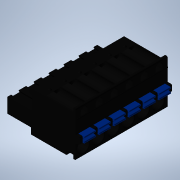
# Autodesk Inventor part: 8079509 6GD-1RR5,08-CLP-CBL
Saved by Autodesk Inventor 2021 (Build 250183000, 183)
## iProperties
Created: 2026-04-23
Part Number: 8079509 6GD-1RR5,08-CLP-CBL
Material: Generic
Catalog Web Link: www.3dfindit.com
Description: NEKM-C6 (p)-terminal strip
Vendor: FESTO
Document SubType Name: Modeling
Designer: psAdmin
Manufacturer: FESTO
Mass: 7.38948 g
Surface Area: 41.4115 cm^2
Volume: 7.38948 cm^3
Density: 1 g/cm^3
Appearance: PSOLRGB-80-80-80
Category: PARTsolutions
Company: FESTO
Title: 8079509 6GD-1RR5,08-CLP-CBL
Author: Cadenas PARTsolutions
Comments: terminal strip
PSOL_IDENT_0: {$CADENAS_DATA/23d-libs/festo/parts/n/nekm/parts/nekm_c6_parts.prj},200 {VTYP=3D},{NB=8079509 6GD-1R
PSOL_IDENT_1: R5,08-CLP-CBL},{LINA=8079509 6GD-1RR5,08-CLP-CBL},{NN=NEKM-C6 (p)},{DATE=26.08.2025 07:05:50},{GEOMD
PSOL_IDENT_2: ATE=26.08.2025 07:05:00},{VERSION=},{LINEID=170},{WBVAR=},{WBNUMERIC=}  {NB=8079509 6GD-1RR5,08-CLP-
PSOL_IDENT_3: CBL},{LINA=8079509 6GD-1RR5,08-CLP-CBL},{KT=DUMMY},{TNR=8079509},{TYP=6GD-1RR5,08-CLP-CBL},{VERS=2},
PSOL_IDENT_4: {N=6},{L=31.100},{L1=3.790}
NB: 8079509 6GD-1RR5,08-CLP-CBL
NN: NEKM-C6 (p)
NT: terminal strip
NBSYN: $TNR. $TYP.
LINA: 8079509 6GD-1RR5,08-CLP-CBL
CATALOG: Festo
TNR: 8079509
TYP: 6GD-1RR5,08-CLP-CBL
VERS: 2
N: 6
L: 31.1
L1: 3.79
SUPPLIER: FESTO
ARTICLENO: 8079509 6GD-1RR5,08-CLP-CBL
BOMINFO: 8079509 6GD-1RR5,08-CLP-CBL
CREATOR: CADENAS GmbH
Autodesk Inventor part; units mm, degrees
sketch "Sketch_1" plane through (0, 0, 0) normal (0, 0, 1) x (1, 0, 0)
  line L0 (0, 6) -> (0, -7.5)
  line L1 (0, -7.5) -> (14.43, -7.5)
  arc A0 (14.43, -7.5) -> (14.73, -7.2) centre (14.43, -7.2) ccw
  line L2 (14.73, -7.2) -> (14.73, 4.1)
  arc A1 (14.73, 4.1) -> (14.73, 4.5) centre (14.73, 4.3) ccw
  line L3 (14.73, 4.5) -> (14.73, 7.2)
  arc A2 (14.73, 7.2) -> (14.43, 7.5) centre (14.43, 7.2) ccw
  line L4 (14.43, 7.5) -> (13.93, 7.5)
  line L5 (13.93, 7.5) -> (13.93, 6)
  line L6 (13.93, 6) -> (0, 6)
  constraints: 14 end point, 6 point on circle, 3 centre point
extrude "Extrusion1" add sketch "Sketch_1" along normal mid plane 31.1
sketch "Sketch_2" plane through (0, 0, 15.55) normal (0, 0, 1) x (1, 0, 0)
  line L0 (14.73, 0.2) -> (14.73, -2.856)
  arc A0 (14.9274, -2.5741) -> (14.73, -2.856) centre (15.03, -2.856) ccw
  line L1 (14.9274, -2.5741) -> (16.0326, -2.1718)
  arc A1 (16.0326, -2.1718) -> (16.23, -1.8899) centre (15.93, -1.8899) ccw
  line L2 (16.23, -1.8899) -> (16.23, -0.3)
  arc A2 (16.23, -0.3) -> (15.93, 0) centre (15.93, -0.3) ccw
  line L3 (15.93, 0) -> (14.93, 0)
  arc A3 (14.73, 0.2) -> (14.93, 0) centre (14.93, 0.2) ccw
  constraints: 8 end point, 8 point on circle, 4 centre point
extrude "Extrusion2" add sketch "Sketch_2" against normal blind 0.8
pattern_linear "Rectangular Pattern1" count 2 spacing 30.3 along (0, 0, -1) of "Extrusion2"
sketch "Sketch_4" plane through (0, 0, 10.65) normal (0, 0, 1) x (1, 0, 0)
  line L0 (14.73, 0.2) -> (14.73, -2.756)
  arc A0 (14.9274, -2.4741) -> (14.73, -2.756) centre (15.03, -2.756) ccw
  line L1 (14.9274, -2.4741) -> (16.0326, -2.0718)
  arc A1 (16.0326, -2.0718) -> (16.23, -1.7899) centre (15.93, -1.7899) ccw
  line L2 (16.23, -1.7899) -> (16.23, -0.3)
  arc A2 (16.23, -0.3) -> (15.93, 0) centre (15.93, -0.3) ccw
  line L3 (15.93, 0) -> (14.93, 0)
  arc A3 (14.73, 0.2) -> (14.93, 0) centre (14.93, 0.2) ccw
  constraints: 8 end point, 8 point on circle, 4 centre point
extrude "Extrusion3" add sketch "Sketch_4" against normal blind 0.98
pattern_linear "Rectangular Pattern2" count 5 spacing 5.08 along (0, 0, -1) of "Extrusion3"
sketch "Sketch_6" plane through (0, 0, 14.65) normal (0, 0, 1) x (1, 0, 0)
  line L0 (14.73, -2.075) -> (16.6, -2.075)
  arc A0 (16.6, -2.075) -> (16.8, -1.875) centre (16.6, -1.875) ccw
  line L1 (16.8, -1.875) -> (16.8, -1.7601)
  arc A1 (16.8, -1.7601) -> (16.6041, -1.516) centre (16.55, -1.7601) ccw
  line L2 (16.6041, -1.516) -> (15.9359, -1.3679)
  arc A2 (15.9359, -0.7821) -> (15.9359, -1.3679) centre (16.0008, -1.075) ccw
  line L3 (15.9359, -0.7821) -> (16.6041, -0.634)
  arc A3 (16.6041, -0.634) -> (16.8, -0.3899) centre (16.55, -0.3899) ccw
  line L4 (16.8, -0.3899) -> (16.8, -0.275)
  arc A4 (16.8, -0.275) -> (16.6, -0.075) centre (16.6, -0.275) ccw
  line L5 (16.6, -0.075) -> (14.73, -0.075)
  line L6 (14.73, -0.075) -> (14.73, -2.075)
  constraints: 14 end point, 10 point on circle, 5 centre point
extrude "Extrusion4" add sketch "Sketch_6" against normal blind 3.9
pattern_linear "Rectangular Pattern3" count 6 spacing 5.08 along (0, 0, -1) of "Extrusion4"
sketch "Sketch_8" plane through (0, -4.65, 0) normal (0, 1, 0) x (1, 0, 0)
  line L0 (14.73, -12.9) -> (11.73, -12.9)
  line L1 (11.73, -12.9) -> (11.73, -10.9)
  line L2 (11.73, -10.9) -> (14.53, -10.9)
  arc A0 (14.53, -10.9) -> (14.73, -10.7) centre (14.53, -10.7) ccw
  line L3 (14.73, -10.7) -> (14.73, -12.9)
  line L4 (14.73, -12.9) -> (11.73, -12.9)
  constraints: 10 end point, 2 point on circle, 1 centre point
revolve "Revolution1" cut sketch "Sketch_8" angle 360 about axis through (14.73, -4.65, 12.9) along (1, 0, 0)
pattern_linear "Rectangular Pattern4" count 6 spacing 5.08 along (0, 0, -1) of "Revolution1"
sketch "Sketch_10" plane through (13.93, 0, 0) normal (1, 0, 0) x (0, 0, -1)
  line L0 (-14.9913, 6) -> (-10.4087, 6)
  arc A0 (-10.4087, 6) -> (-14.9913, 6) centre (-12.7, 5) ccw
  constraints: 2 end point, 2 point on circle, 1 centre point
extrude "Extrusion5" add sketch "Sketch_10" against normal blind 9.7
pattern_linear "Rectangular Pattern5" count 6 spacing 5.08 along (0, 0, -1) of "Extrusion5"
sketch "Sketch_12" plane through (0, 0, 0) normal (0, 0, 1) x (1, 0, 0)
  line L0 (2, 7.5) -> (2, 6)
  line L1 (2, 6) -> (4.23, 6)
  line L2 (4.23, 6) -> (5.73, 7.5)
  line L3 (5.73, 7.5) -> (2, 7.5)
  constraints: 8 end point
extrude "Extrusion6" cut sketch "Sketch_12" along normal mid plane 31.1
sketch "Sketch_13" plane through (14.73, 0, 0) normal (1, 0, 0) x (0, 0, -1)
  line L0 (-13.875, 5.775) -> (-13.875, 4.6)
  line L1 (-13.875, 4.6) -> (-11.525, 4.6)
  line L2 (-11.525, 4.6) -> (-11.525, 5.775)
  arc A0 (-11.525, 5.775) -> (-13.875, 5.775) centre (-12.7, 5.775) ccw
  constraints: 6 end point, 2 point on circle, 1 centre point
extrude "Extrusion7" cut sketch "Sketch_13" against normal blind 9.325
pattern_linear "Rectangular Pattern6" count 6 spacing 5.08 along (0, 0, -1) of "Extrusion7"
sketch "Sketch_15" plane through (0, 7.5, 0) normal (0, 1, 0) x (1, 0, 0)
  arc A0 (5.405, -11.525) -> (5.405, -13.875) centre (5.405, -12.7) ccw
  line L0 (5.405, -13.875) -> (6.58, -13.875)
  line L1 (6.58, -13.875) -> (6.58, -11.525)
  line L2 (6.58, -11.525) -> (5.405, -11.525)
  constraints: 6 end point, 2 point on circle, 1 centre point
extrude "Extrusion8" cut sketch "Sketch_15" against normal blind 2.9
pattern_linear "Rectangular Pattern7" count 6 spacing 5.08 along (0, 0, -1) of "Extrusion8"
sketch "Sketch_17" plane through (3.13, 0, 0) normal (1, 0, 0) x (0, 0, -1)
  line L0 (-12.7, 6) -> (-12.7, 6.3)
  arc A0 (-12.25, 6) -> (-12.7, 6.3) centre (-12.7083, 5.8001) ccw
  line L1 (-12.25, 6) -> (-12.7, 6)
  line L2 (-12.7, 6) -> (-12.7, 6.3)
  constraints: 6 end point, 2 point on circle, 1 centre point
revolve "Revolution2" add sketch "Sketch_17" angle 360 about axis through (3.13, 6, 12.7) along (0, -1, 0)
pattern_linear "Rectangular Pattern8" count 6 spacing 5.08 along (0, 0, -1) of "Revolution2"
sketch "Sketch_25" plane through (0, 0, 0) normal (0, 0, 1) x (1, 0, 0)
  line L0 (-0.5, -0.795) -> (-0.5, -7.5)
  line L1 (-0.5, -7.5) -> (0, -7.5)
  line L2 (0, -7.5) -> (0, 0.071)
  line L3 (0, 0.071) -> (-0.5, -0.795)
  constraints: 8 end point
extrude "Extrusion9" add sketch "Sketch_25" along normal mid plane 31.1
sketch "Sketch_37" plane through (-0.5, 0, 0) normal (1, 0, 0) x (0, 0, -1)
  line L0 (-15.24, -5.71) -> (-14.8207, -5.71)
  arc A0 (-14.8207, -5.71) -> (-10.5793, -5.71) centre (-12.7, -3.71) ccw
  line L1 (-10.5793, -5.71) -> (-9.7407, -5.71)
  arc A1 (-9.7407, -5.71) -> (-5.4993, -5.71) centre (-7.62, -3.71) ccw
  line L2 (-5.4993, -5.71) -> (-4.6607, -5.71)
  arc A2 (-4.6607, -5.71) -> (-0.4193, -5.71) centre (-2.54, -3.71) ccw
  line L3 (-0.4193, -5.71) -> (0.4193, -5.71)
  arc A3 (0.4193, -5.71) -> (4.6607, -5.71) centre (2.54, -3.71) ccw
  line L4 (4.6607, -5.71) -> (5.4993, -5.71)
  arc A4 (5.4993, -5.71) -> (9.7407, -5.71) centre (7.62, -3.71) ccw
  line L5 (9.7407, -5.71) -> (10.5793, -5.71)
  arc A5 (10.5793, -5.71) -> (14.8207, -5.71) centre (12.7, -3.71) ccw
  line L6 (14.8207, -5.71) -> (15.24, -5.71)
  line L7 (15.24, -5.71) -> (15.24, -0.795)
  line L8 (15.24, -0.795) -> (13.957, -0.795)
  line L9 (13.957, -0.795) -> (14.3496, -1.475)
  line L10 (14.3496, -1.475) -> (11.0534, -1.475)
  line L11 (11.0534, -1.475) -> (11.446, -0.795)
  line L12 (11.446, -0.795) -> (8.877, -0.795)
  line L13 (8.877, -0.795) -> (9.2696, -1.475)
  line L14 (9.2696, -1.475) -> (5.9734, -1.475)
  line L15 (5.9734, -1.475) -> (6.366, -0.795)
  line L16 (6.366, -0.795) -> (3.797, -0.795)
  line L17 (3.797, -0.795) -> (4.1896, -1.475)
  line L18 (4.1896, -1.475) -> (0.8934, -1.475)
  line L19 (0.8934, -1.475) -> (1.286, -0.795)
  line L20 (1.286, -0.795) -> (-1.283, -0.795)
  line L21 (-1.283, -0.795) -> (-0.8904, -1.475)
  line L22 (-0.8904, -1.475) -> (-4.1866, -1.475)
  line L23 (-4.1866, -1.475) -> (-3.794, -0.795)
  line L24 (-3.794, -0.795) -> (-6.363, -0.795)
  line L25 (-6.363, -0.795) -> (-5.9704, -1.475)
  line L26 (-5.9704, -1.475) -> (-9.2666, -1.475)
  line L27 (-9.2666, -1.475) -> (-8.874, -0.795)
  line L28 (-8.874, -0.795) -> (-11.443, -0.795)
  line L29 (-11.443, -0.795) -> (-11.0504, -1.475)
  line L30 (-11.0504, -1.475) -> (-14.3466, -1.475)
  line L31 (-14.3466, -1.475) -> (-13.954, -0.795)
  line L32 (-13.954, -0.795) -> (-15.24, -0.795)
  line L33 (-15.24, -0.795) -> (-15.24, -5.71)
  constraints: 68 end point, 12 point on circle, 6 centre point
extrude "Extrusion10" add sketch "Sketch_37" against normal blind 8.3
sketch "Sketch13" plane through (-8.8, 0, 0) normal (-1, 0, 0) x (0, 0, 1)
  point P0 (12.7, -3.71)
hole "Hole1" at (-8.8, -3.71, 12.7) direction (1, 0, 0) diameter 1.4 depth 2 counterbore diameter 2.8 counterbore depth 1
pattern_linear "Rectangular Pattern9" count 6 spacing 5.08 along (0, 0, -1) of "Hole1"
sketch "Sketch_30" plane through (0, 0, 11.76) normal (0, 0, 1) x (1, 0, 0)
  arc A0 (-4.9014, 1.2616) -> (-4.86, 0.947) centre (-4.76, 1.1202) ccw
  line L0 (-4.86, 0.947) -> (-4.1642, 0.5453)
  arc A1 (-4.1642, 0.5453) -> (-3.8021, 0.5929) centre (-4.0142, 0.8051) ccw
  line L1 (-3.8021, 0.5929) -> (-3.53, 0.865)
  line L2 (-3.53, 0.865) -> (-0.3256, 1.0049)
  arc A2 (-0.3, 0.406) -> (-0.3256, 1.0049) centre (-0.3, 0.706) ccw
  arc A3 (-0.3, 0.406) -> (-0.5, 0.206) centre (-0.3, 0.206) ccw
  line L3 (-0.5, 0.206) -> (-0.5, -1)
  line L4 (-0.5, -1) -> (0.5, -1)
  line L5 (0.5, -1) -> (0.5, 3.3534)
  line L6 (0.5, 3.3534) -> (0, 3.3534)
  arc A4 (-0.2325, 3.0611) -> (0, 3.3534) centre (-0.3, 3.3534) ccw
  line L7 (-0.2325, 3.0611) -> (-3.7536, 2.2482)
  arc A5 (-3.7536, 2.2482) -> (-4.1152, 2.0478) centre (-3.5849, 1.5174) ccw
  line L8 (-4.1152, 2.0478) -> (-4.9014, 1.2616)
  constraints: 18 end point, 12 point on circle, 6 centre point
extrude "Extrusion11" add sketch "Sketch_30" against normal blind 1.6
sketch "Sketch_31" plane through (0, 0, -11.76) normal (0, 0, 1) x (1, 0, 0)
  arc A0 (-4.9014, 1.2616) -> (-4.86, 0.947) centre (-4.76, 1.1202) ccw
  line L0 (-4.86, 0.947) -> (-4.1642, 0.5453)
  arc A1 (-4.1642, 0.5453) -> (-3.8021, 0.5929) centre (-4.0142, 0.8051) ccw
  line L1 (-3.8021, 0.5929) -> (-3.53, 0.865)
  line L2 (-3.53, 0.865) -> (-0.3256, 1.0049)
  arc A2 (-0.3, 0.406) -> (-0.3256, 1.0049) centre (-0.3, 0.706) ccw
  arc A3 (-0.3, 0.406) -> (-0.5, 0.206) centre (-0.3, 0.206) ccw
  line L3 (-0.5, 0.206) -> (-0.5, -1)
  line L4 (-0.5, -1) -> (0.5, -1)
  line L5 (0.5, -1) -> (0.5, 3.3534)
  line L6 (0.5, 3.3534) -> (0, 3.3534)
  arc A4 (-0.2325, 3.0611) -> (0, 3.3534) centre (-0.3, 3.3534) ccw
  line L7 (-0.2325, 3.0611) -> (-3.7536, 2.2482)
  arc A5 (-3.7536, 2.2482) -> (-4.1152, 2.0478) centre (-3.5849, 1.5174) ccw
  line L8 (-4.1152, 2.0478) -> (-4.9014, 1.2616)
  constraints: 18 end point, 12 point on circle, 6 centre point
extrude "Extrusion12" add sketch "Sketch_31" along normal blind 1.6
sketch "Sketch_39" plane through (11.58, 0, 0) normal (1, 0, 0) x (0, 0, -1)
  line L0 (-15.55, -8.25) -> (15.55, -8.25)
  line L1 (15.55, -8.25) -> (15.55, -6.25)
  line L2 (15.55, -6.25) -> (14.8585, -6.25)
  arc A0 (10.1415, -6.25) -> (14.8585, -6.25) centre (12.5, -4.65) ccw
  line L3 (10.1415, -6.25) -> (9.7785, -6.25)
  arc A1 (5.0615, -6.25) -> (9.7785, -6.25) centre (7.42, -4.65) ccw
  line L4 (5.0615, -6.25) -> (4.6985, -6.25)
  arc A2 (-0.0185, -6.25) -> (4.6985, -6.25) centre (2.34, -4.65) ccw
  line L5 (-0.0185, -6.25) -> (-0.3815, -6.25)
  arc A3 (-5.0985, -6.25) -> (-0.3815, -6.25) centre (-2.74, -4.65) ccw
  line L6 (-5.0985, -6.25) -> (-5.4615, -6.25)
  arc A4 (-10.1785, -6.25) -> (-5.4615, -6.25) centre (-7.82, -4.65) ccw
  line L7 (-10.1785, -6.25) -> (-10.5415, -6.25)
  arc A5 (-15.2585, -6.25) -> (-10.5415, -6.25) centre (-12.9, -4.65) ccw
  line L8 (-15.2585, -6.25) -> (-15.55, -6.25)
  line L9 (-15.55, -6.25) -> (-15.55, -8.25)
  constraints: 20 end point, 12 point on circle, 6 centre point
extrude "Extrusion13" cut sketch "Sketch_39" along normal blind 2.35
ref_plane "ANBAU_XY" through (0, 0, 0) normal (0, 1, 0) x (1, 0, 0)
ref_plane "ANBAU_YZ" through (0, 0, 0) normal (1, 0, 0) x (0, 0, -1)
ref_plane "ANBAU_ZX" through (0, 0, 0) normal (0, 0, -1) x (0, 1, 0)
ref_plane "CP1_XY" through (-0.5, -3.71, 0) normal (1, 0, 0) x (0, 0, -1)
ref_plane "CP1_YZ" through (-0.5, -3.71, 0) normal (0, 0, -1) x (0, 1, 0)
ref_plane "CP1_ZX" through (-0.5, -3.71, 0) normal (0, 1, 0) x (1, 0, 0)
ref_plane "ECP_1_XY" through (2.73, -4.65, 12.9) normal (1, 0, 0) x (0, 0, -1)
ref_plane "ECP_1_YZ" through (2.73, -4.65, 12.9) normal (0, 0, -1) x (0, 1, 0)
ref_plane "ECP_1_ZX" through (2.73, -4.65, 12.9) normal (0, 1, 0) x (1, 0, 0)
ref_plane "ECP_2_XY" through (2.73, -4.65, 7.82) normal (1, 0, 0) x (0, 0, -1)
ref_plane "ECP_2_YZ" through (2.73, -4.65, 7.82) normal (0, 0, -1) x (0, 1, 0)
ref_plane "ECP_2_ZX" through (2.73, -4.65, 7.82) normal (0, 1, 0) x (1, 0, 0)
ref_plane "ECP_3_XY" through (2.73, -4.65, 2.74) normal (1, 0, 0) x (0, 0, -1)
ref_plane "ECP_3_YZ" through (2.73, -4.65, 2.74) normal (0, 0, -1) x (0, 1, 0)
ref_plane "ECP_3_ZX" through (2.73, -4.65, 2.74) normal (0, 1, 0) x (1, 0, 0)
ref_plane "ECP_4_XY" through (2.73, -4.65, -2.34) normal (1, 0, 0) x (0, 0, -1)
ref_plane "ECP_4_YZ" through (2.73, -4.65, -2.34) normal (0, 0, -1) x (0, 1, 0)
ref_plane "ECP_4_ZX" through (2.73, -4.65, -2.34) normal (0, 1, 0) x (1, 0, 0)
ref_plane "ECP_5_XY" through (2.73, -4.65, -7.42) normal (1, 0, 0) x (0, 0, -1)
ref_plane "ECP_5_YZ" through (2.73, -4.65, -7.42) normal (0, 0, -1) x (0, 1, 0)
ref_plane "ECP_5_ZX" through (2.73, -4.65, -7.42) normal (0, 1, 0) x (1, 0, 0)
ref_plane "ECP_6_XY" through (2.73, -4.65, -12.5) normal (1, 0, 0) x (0, 0, -1)
ref_plane "ECP_6_YZ" through (2.73, -4.65, -12.5) normal (0, 0, -1) x (0, 1, 0)
ref_plane "ECP_6_ZX" through (2.73, -4.65, -12.5) normal (0, 1, 0) x (1, 0, 0)
ref_plane "MD_XY" through (-8.8, -3.71, 12.7) normal (-1, 0, 0) x (0, 0, -1)
ref_plane "MD_YZ" through (-8.8, -3.71, 12.7) normal (0, 0, -1) x (0, -1, 0)
ref_plane "MD_ZX" through (-8.8, -3.71, 12.7) normal (0, -1, 0) x (-1, 0, 0)
ref_plane "OP_XY" through (-8.8, 7.5, -15.55) normal (1, 0, 0) x (0, 0, 1)
ref_plane "OP_YZ" through (-8.8, 7.5, -15.55) normal (0, 0, 1) x (0, -1, 0)
ref_plane "OP_ZX" through (-8.8, 7.5, -15.55) normal (0, -1, 0) x (1, 0, 0)
body "Solid1"
